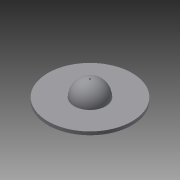
# Autodesk Inventor part: flower
Saved by Autodesk Inventor 2014 (Build 180170000, 170)
## iProperties
Created: 2014-04-02
Part Number: flower
Material: Generic
Document SubType Name: Modeling
Designer: jferner
Density: 1 g/cm^3
Appearance: Default
Author: jferner
Autodesk Inventor part; units mm, degrees
ref_plane "YZ Plane" through (0, 0, 0) normal (1, 0, 0) x (0, 1, 0)
ref_plane "XZ Plane" through (0, 0, 0) normal (0, 1, 0) x (-1, 0, 0)
ref_plane "XY Plane" through (0, 0, 0) normal (0, 0, 1) x (1, 0, 0)
sketch "Sketch1" plane through (0, 0, 0) normal (0, 1, 0) x (-1, 0, 0)
  circle A0 centre (0, 0) radius 25.4
  dimension "d0" = 50.8
  constraints: 1 centre point, 1 coincident
  measures "d0" diameter of A0
extrude "Extrusion1" add sketch "Sketch1" along normal blind 2
sketch "Sketch3" plane through (0, 0, 0) normal (0, 0, 1) x (1, 0, 0)
  line L0 (-25.4, 0) -> (25.4, 0) projected
  line L1 (25.4, 2) -> (-25.4, 2) projected
  line L2 (0, 2) -> (0, 13.4486)
  arc A0 (9.3127, 0) -> (9.525, 2) centre (0, 2) ccw
  arc A1 (0, 11.525) -> (-9.3127, 0) centre (0, 2) ccw
  line L3 (0, 2) -> (-9.525, 2)
  point P0 (0, 0)
  constraints: 5 point on circle, 5 point on line, 4 end point, 2 centre point, 1 midpoint, 1 perpendicular
revolve "Revolution1" add sketch "Sketch3" angle 360 about axis through (0, 2, 0) along (0, 1, 0) contours A1 L2 L1
sketch "Sketch2" plane through (0, 2, 0) normal (0, 1, 0) x (1, 0, 0)
  circle A0 centre (0, 0) radius 25.4 projected
  circle A1 centre (0, 0) radius 0.5
  dimension "d3" = 1
  constraints: 1 centre point, 1 coincident
  measures "d3" diameter of A1
extrude "Extrusion2" cut sketch "Sketch2" along normal through all both and the other way through all contours A1
body "Solid1"
